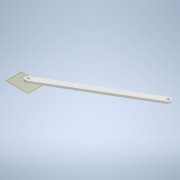
# Autodesk Inventor part: truss final piece
Saved by Autodesk Inventor 2020 (Build 240168000, 168)
## iProperties
Created: 2020-07-04
Part Number: truss final piece
Material: Generic
Document SubType Name: Modeling
Designer: Ashiqrahman
Density: 1 g/cm^3
Appearance: Default
Author: Ashiqrahman
Autodesk Inventor part; units mm, degrees
ref_plane "YZ Plane" through (0, 0, 0) normal (1, 0, 0) x (0, 1, 0)
ref_plane "XZ Plane" through (0, 0, 0) normal (0, 1, 0) x (-1, 0, 0)
ref_plane "XY Plane" through (0, 0, 0) normal (0, 0, 1) x (1, 0, 0)
ref_plane "Work Plane1" through (-47.4023, 137.8054, 11.1867) normal (0, 1, 0) x (-1, 0, 0)
sketch "Sketch1" plane through (-47.4023, 137.8054, 11.1867) normal (0, 1, 0) x (-1, 0, 0)
  line L0 (13.9385, 9.5711) -> (4.3301, -7.0711) projected
  line L1 (-13.9385, 9.5711) -> (13.9385, 9.5711) projected
  line L2 (-4.3301, -7.0711) -> (-13.9385, 9.5711) projected
  arc A0 (-4.3301, -7.0711) -> (4.3301, -7.0711) centre (0, -4.5711) ccw projected
  circle A1 centre (0, -4.5711) radius 2 projected
  line L3 (-115.8579, -75.4289) -> (-115.8579, -90.4289) projected
  arc A2 (-115.8579, -75.4289) -> (-120.8579, -70.4289) centre (-120.8579, -75.4289) ccw projected
  line L4 (-135.8579, -70.4289) -> (-120.8579, -70.4289) projected
  line L5 (-135.8579, -90.4289) -> (-135.8579, -70.4289) projected
  line L6 (-115.8579, -90.4289) -> (-135.8579, -90.4289) projected
  circle A3 centre (-121.7157, -76.2868) radius 2 projected
  line L7 (-121.7157, -76.2868) -> (0, -4.5711) construction
  line L8 (-119.6852, -79.7331) -> (2.0306, -8.0173)
  line L9 (-2.0306, -1.1248) -> (-123.7463, -72.8405)
  arc A4 (-123.7463, -72.8405) -> (-119.6852, -79.7331) centre (-121.7157, -76.2868) ccw
  arc A5 (2.0306, -8.0173) -> (-2.0306, -1.1248) centre (0, -4.5711) ccw
  point P0 (-47.4023, -11.1867)
  point P1 (-60.8579, -40.4289)
  dimension "d0" = 8
  constraints: 8 end point, 4 point on circle, 4 tangent, 2 centre point, 1 midpoint, 1 parallel
  measures "d0" diameter of A5
extrude "Extrusion1" add sketch "Sketch1" along normal blind 3 contours L8 L3 A2 L9 L2 A0 | A0 L2 L9 A5 L8 | L8 A4 L9 A2 L3
body "Solid1"
